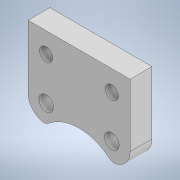
# Autodesk Inventor part: upper slider pen
Saved by Autodesk Inventor 2020 (Build 240168000, 168)
## iProperties
Created: 2026-07-08
Part Number: upper slider pen
Material: Generic
Document SubType Name: Modeling
Designer: drago
Density: 1 g/cm^3
Appearance: Default
Author: drago
Autodesk Inventor part; units mm, degrees
ref_plane "YZ Plane" through (0, 0, 0) normal (1, 0, 0) x (0, 1, 0)
ref_plane "XZ Plane" through (0, 0, 0) normal (0, 1, 0) x (-1, 0, 0)
ref_plane "XY Plane" through (0, 0, 0) normal (0, 0, 1) x (1, 0, 0)
sketch "Sketch1" plane through (0, 0, 0) normal (0, 0, 1) x (1, 0, 0)
  line L0 (7, -20) -> (7, -17)
  line L1 (-7, -17) -> (7, -17)
  line L2 (-7, -17) -> (-7, -20)
  arc A0 (-7, -20) -> (-4.5, -22.5) centre (-4.5, -20) ccw
  line L3 (-4.5, -22.5) -> (4.5, -22.5)
  arc A1 (4.5, -22.5) -> (7, -20) centre (4.5, -20) ccw
  circle A2 centre (-4.5, -20) radius 1
  circle A3 centre (4.5, -20) radius 1
  line L4 (7, -11.4) -> (-7, -11.4)
  line L5 (-7, -11.4) -> (-7, -17)
  line L6 (-7, -17) -> (7, -17)
  line L7 (7, -17) -> (7, -11.4)
  circle A4 centre (4.5, -14.2) radius 0.9
  circle A5 centre (-4.5, -14.2) radius 0.9
  point P0 (0, 0)
  constraints: 16 end point, 6 centre point, 4 point on circle
extrude "Extrusion1" add sketch "Sketch1" along normal blind 3
sketch "Sketch2" plane through (0, 0, 3) normal (0, 0, 1) x (1, 0, 0)
  circle A0 centre (-4.5, -20) radius 1 projected
  circle A1 centre (4.5, -20) radius 1 projected
  circle A2 centre (0, -27.2111) radius 6.5
  point P0 (0, 0)
  constraints: 1 centre point
extrude "Extrusion2" cut sketch "Sketch2" against normal blind 3 contours A2
fillet "Fillet1" radius 1 2 edges at (-4.4783, -22.5, 1.5) (4.4783, -22.5, 1.5)
body "Solid1"
